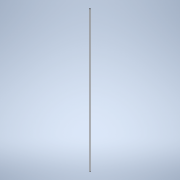
# Autodesk Inventor part: wand
Saved by Autodesk Inventor 2021 (Build 250183000, 183)
## iProperties
Created: 2021-03-29
Part Number: wand
Material: Stainless Steel
Document SubType Name: Modeling
Designer: Work
Mass: 809.335 g
Surface Area: 1226.67 cm^2
Volume: 101.167 cm^3
Density: 8 g/cm^3
Appearance: Semi-Polished
Author: Work
Autodesk Inventor part; units mm, degrees
ref_plane "YZ Plane" through (0, 0, 0) normal (1, 0, 0) x (0, 1, 0)
ref_plane "XZ Plane" through (0, 0, 0) normal (0, 1, 0) x (-1, 0, 0)
ref_plane "XY Plane" through (0, 0, 0) normal (0, 0, 1) x (1, 0, 0)
sketch "Sketch1" plane through (0, 0, 0) normal (0, 1, 0) x (-1, 0, 0)
  circle A0 centre (0, 0) radius 4.699
  circle A1 centre (0, 0) radius 6.35
  dimension "d2" = 9.398
  dimension "d3" = 12.7
  constraints: 2 centre point, 2 coincident
  measures "d2" diameter of A0
  measures "d3" diameter of A1
extrude "Extrusion1" add sketch "Sketch1" along normal blind 1765.3
body "Solid1"
